Autodesk Inventor part; units mm, degrees
(part 2 of 2)
sketch "Sketch8" plane through (0, 0, 0) normal (0, 0, -1) x (-1, 0, 0)
  arc A0 (-1.4446, 6.1835) -> (1.4446, 6.1835) centre (0, 0) ccw construction
  circle A1 centre (0, 0) radius 44.45 construction
  spline S0 degree 2 poles (9.5387, -40.7098) (10.0629, -40.5828) (11.0086, -40.6927) (11.3992, -40.9412) knots 0 0 0 1 2 2 2
  spline S1 degree 2 poles (11.3992, -40.9412) (11.7907, -41.1937) (12.3573, -42.0815) (12.5094, -42.7097) knots 0 0 0 1 2 2 2
  spline S2 degree 2 poles (12.5094, -42.7097) (12.6538, -43.3058) (12.5463, -44.3315) (12.3156, -44.7431) knots 0 0 0 1 2 2 2
  spline S3 degree 2 poles (12.3156, -44.7431) (12.094, -45.1399) (11.2991, -45.7052) (10.7749, -45.8321) knots 0 0 0 1 2 2 2
  spline S4 degree 2 poles (10.7749, -45.8321) (10.5229, -45.8931) (10.0493, -45.9316) (9.8258, -45.9179) knots 0 0 0 1 2 2 2
  spline S5 degree 2 poles (9.8258, -45.9179) (9.6461, -45.9106) (9.1954, -45.8334) (9.0558, -45.7994) knots 0 0 0 1 2 2 2
  line L0 (9.0558, -45.7994) -> (8.864, -45.0072)
  line L1 (8.864, -45.0072) -> (8.92, -44.9936)
  spline S6 degree 2 poles (8.92, -44.9936) (9.0702, -45.0716) (9.3777, -45.2047) (9.6449, -45.2586) knots 0 0 0 1 2 2 2
  spline S7 degree 2 poles (9.6449, -45.2586) (9.8692, -45.3102) (10.4173, -45.3172) (10.7134, -45.2455) knots 0 0 0 1 2 2 2
  spline S8 degree 2 poles (10.7134, -45.2455) (11.4256, -45.0731) (12.0461, -43.7876) (11.8301, -42.8954) knots 0 0 0 1 2 2 2
  spline S9 degree 2 poles (11.8301, -42.8954) (11.7099, -42.3992) (11.2976, -41.7113) (11.0156, -41.5085) knots 0 0 0 1 2 2 2
  spline S10 degree 2 poles (11.0156, -41.5085) (10.7415, -41.3038) (10.0764, -41.181) (9.7003, -41.2721) knots 0 0 0 1 2 2 2
  spline S11 degree 2 poles (9.7003, -41.2721) (9.4243, -41.339) (8.8915, -41.5527) (8.7228, -41.6783) knots 0 0 0 1 2 2 2
  line L2 (8.7228, -41.6783) -> (9.0319, -42.9546)
  line L3 (9.0319, -42.9546) -> (10.1762, -42.6775)
  line L4 (10.1762, -42.6775) -> (10.3157, -43.2536)
  line L5 (10.3157, -43.2536) -> (8.5233, -43.6877)
  line L6 (8.5233, -43.6877) -> (8.001, -41.5311)
  spline S12 degree 2 poles (8.001, -41.5311) (8.1115, -41.4451) (8.4939, -41.1703) (8.6614, -41.0747) knots 0 0 0 1 2 2 2
  spline S13 degree 2 poles (8.6614, -41.0747) (8.888, -40.9436) (9.2627, -40.7766) (9.5387, -40.7098) knots 0 0 0 1 2 2 2
  spline S14 degree 2 poles (5.4812, -41.4638) (6.3864, -41.3379) (7.5225, -42.2148) (7.6529, -43.1527) knots 0 0 0 1 2 2 2
  spline S15 degree 2 poles (7.6529, -43.1527) (7.7811, -44.0742) (6.9667, -45.3013) (6.1879, -45.4096) knots 0 0 0 1 2 2 2
  spline S16 degree 2 poles (6.1879, -45.4096) (5.8372, -45.4584) (5.2666, -45.3299) (5.0367, -45.1416) knots 0 0 0 1 2 2 2
  spline S17 degree 2 poles (5.0367, -45.1416) (4.8028, -44.9538) (4.4999, -44.36) (4.437, -43.9074) knots 0 0 0 1 2 2 2
  line L7 (4.437, -43.9074) -> (4.3888, -43.5608)
  line L8 (4.3888, -43.5608) -> (7.0024, -43.1974)
  spline S18 degree 2 poles (7.0024, -43.1974) (6.9112, -42.5409) (6.1537, -41.9355) (5.5665, -42.0172) knots 0 0 0 1 2 2 2
  spline S19 degree 2 poles (5.5665, -42.0172) (5.3585, -42.0461) (4.9679, -42.196) (4.815, -42.2921) knots 0 0 0 1 2 2 2
  spline S20 degree 2 poles (4.815, -42.2921) (4.6551, -42.3974) (4.4385, -42.573) (4.3701, -42.6491) knots 0 0 0 1 2 2 2
  line L9 (4.3701, -42.6491) -> (4.3334, -42.6542)
  line L10 (4.3334, -42.6542) -> (4.237, -41.961)
  spline S21 degree 2 poles (4.237, -41.961) (4.3408, -41.9008) (4.657, -41.7239) (4.7824, -41.669) knots 0 0 0 1 2 2 2
  spline S22 degree 2 poles (4.7824, -41.669) (4.9585, -41.5905) (5.2529, -41.4955) (5.4812, -41.4638) knots 0 0 0 1 2 2 2
  spline S23 degree 2 poles (5.076, -43.9599) (5.1199, -44.2156) (5.2781, -44.576) (5.3976, -44.6882) knots 0 0 0 1 2 2 2
  spline S24 degree 2 poles (5.3976, -44.6882) (5.5276, -44.8156) (5.8951, -44.9183) (6.152, -44.8826) knots 0 0 0 1 2 2 2
  spline S25 degree 2 poles (6.152, -44.8826) (6.4048, -44.8474) (6.7386, -44.6472) (6.8649, -44.48) knots 0 0 0 1 2 2 2
  spline S26 degree 2 poles (6.8649, -44.48) (6.9867, -44.3093) (7.083, -43.926) (7.0699, -43.6826) knots 0 0 0 1 2 2 2
  line L11 (7.0699, -43.6826) -> (5.076, -43.9599)
  spline S27 degree 2 poles (1.3862, -42.2975) (1.4614, -42.236) (1.7141, -42.0171) (1.8343, -41.9491) knots 0 0 0 1 2 2 2
  spline S28 degree 2 poles (1.8343, -41.9491) (1.9983, -41.8501) (2.3101, -41.7395) (2.5979, -41.725) knots 0 0 0 1 2 2 2
  spline S29 degree 2 poles (2.5979, -41.725) (2.8322, -41.7131) (3.2647, -41.8684) (3.4331, -42.0207) knots 0 0 0 1 2 2 2
  spline S30 degree 2 poles (3.4331, -42.0207) (3.5932, -42.1692) (3.8015, -42.6203) (3.8144, -42.8752) knots 0 0 0 1 2 2 2
  spline S31 degree 2 poles (3.8144, -42.8752) (3.8344, -43.2699) (3.5297, -43.8459) (3.176, -44.0246) knots 0 0 0 1 2 2 2
  spline S32 degree 2 poles (3.176, -44.0246) (2.8628, -44.1889) (1.9968, -44.344) (1.4926, -44.3984) knots 0 0 0 1 2 2 2
  line L12 (1.4926, -44.3984) -> (1.4988, -44.5218)
  spline S33 degree 2 poles (1.4988, -44.5218) (1.5101, -44.7438) (1.6597, -45.0124) (1.787, -45.0842) knots 0 0 0 1 2 2 2
  spline S34 degree 2 poles (1.787, -45.0842) (1.9143, -45.1561) (2.2704, -45.1875) (2.4595, -45.1779) knots 0 0 0 1 2 2 2
  spline S35 degree 2 poles (2.4595, -45.1779) (2.6815, -45.1667) (3.2751, -45.0047) (3.5688, -44.8621) knots 0 0 0 1 2 2 2
  line L13 (3.5688, -44.8621) -> (3.6058, -44.8602)
  line L14 (3.6058, -44.8602) -> (3.6389, -45.5139)
  spline S36 degree 2 poles (3.6389, -45.5139) (3.4646, -45.5722) (2.809, -45.7291) (2.4841, -45.7455) knots 0 0 0 1 2 2 2
  spline S37 degree 2 poles (2.4841, -45.7455) (2.0895, -45.7655) (1.5446, -45.6695) (1.3227, -45.5199) knots 0 0 0 1 2 2 2
  spline S38 degree 2 poles (1.3227, -45.5199) (1.1051, -45.3743) (0.8743, -44.8873) (0.8562, -44.5296) knots 0 0 0 1 2 2 2
  line L15 (0.8562, -44.5296) -> (0.7244, -41.927)
  line L16 (0.7244, -41.927) -> (1.3658, -41.8946)
  line L17 (1.3658, -41.8946) -> (1.3862, -42.2975)
  line L18 (1.4132, -42.832) -> (1.4668, -43.8886)
  spline S39 degree 2 poles (1.4668, -43.8886) (1.696, -43.8564) (2.3873, -43.7513) (2.6018, -43.6745) knots 0 0 0 1 2 2 2
  spline S40 degree 2 poles (2.6018, -43.6745) (2.8528, -43.5834) (3.1693, -43.2418) (3.1548, -42.954) knots 0 0 0 1 2 2 2
  spline S41 degree 2 poles (3.1548, -42.954) (3.1381, -42.625) (2.7512, -42.3108) (2.3976, -42.3287) knots 0 0 0 1 2 2 2
  spline S42 degree 2 poles (2.3976, -42.3287) (2.0975, -42.3439) (1.6172, -42.6279) (1.4132, -42.832) knots 0 0 0 1 2 2 2
  line L19 (-2.2698, -44.9941) -> (-2.2369, -44.9948)
  spline S43 degree 2 poles (-2.2369, -44.9948) (-2.1633, -45.0171) (-2.0029, -45.0291) (-1.8918, -45.0316) knots 0 0 0 1 2 2 2
  spline S44 degree 2 poles (-1.8918, -45.0316) (-1.6325, -45.0377) (-1.117, -44.8231) (-0.8813, -44.6062) knots 0 0 0 1 2 2 2
  line L20 (-0.8813, -44.6062) -> (-0.8187, -41.9023)
  line L21 (-0.8187, -41.9023) -> (-0.1766, -41.9172)
  line L22 (-0.1766, -41.9172) -> (-0.265, -45.7282)
  line L23 (-0.265, -45.7282) -> (-0.907, -45.7133)
  line L24 (-0.907, -45.7133) -> (-0.8938, -45.1454)
  spline S45 degree 2 poles (-0.8938, -45.1454) (-1.2509, -45.45) (-1.7795, -45.6931) (-2.0264, -45.6874) knots 0 0 0 1 2 2 2
  spline S46 degree 2 poles (-2.0264, -45.6874) (-2.1252, -45.6851) (-2.2238, -45.6746) (-2.2852, -45.6608) knots 0 0 0 1 2 2 2
  line L25 (-2.2852, -45.6608) -> (-2.2698, -44.9941)
  line L26 (-8.8009, -41.0388) -> (-7.9348, -41.1759)
  line L27 (-7.9348, -41.1759) -> (-6.6649, -43.4233)
  line L28 (-6.6649, -43.4233) -> (-5.9005, -43.5442)
  line L29 (-5.9005, -43.5442) -> (-5.5846, -41.5478)
  line L30 (-5.5846, -41.5478) -> (-4.9177, -41.6533)
  line L31 (-4.9177, -41.6533) -> (-5.7117, -46.6709)
  line L32 (-5.7117, -46.6709) -> (-7.0047, -46.4662)
  spline S47 degree 2 poles (-7.0047, -46.4662) (-7.4357, -46.398) (-8.0024, -46.2125) (-8.2397, -45.9999) knots 0 0 0 1 2 2 2
  spline S48 degree 2 poles (-8.2397, -45.9999) (-8.4769, -45.7873) (-8.6976, -45.2064) (-8.6352, -44.812) knots 0 0 0 1 2 2 2
  spline S49 degree 2 poles (-8.6352, -44.812) (-8.5483, -44.2631) (-7.8695, -43.6078) (-7.3613, -43.5048) knots 0 0 0 1 2 2 2
  line L33 (-7.3613, -43.5048) -> (-8.8009, -41.0388)
  spline S50 degree 2 poles (-7.9315, -44.8692) (-7.9663, -45.0887) (-7.8652, -45.4507) (-7.7199, -45.5862) knots 0 0 0 1 2 2 2
  spline S51 degree 2 poles (-7.7199, -45.5862) (-7.5924, -45.7022) (-7.2264, -45.8393) (-6.9499, -45.8831) knots 0 0 0 1 2 2 2
  line L34 (-6.9499, -45.8831) -> (-6.2872, -45.9879)
  line L35 (-6.2872, -45.9879) -> (-5.9886, -44.1013)
  line L36 (-5.9886, -44.1013) -> (-6.5741, -44.0086)
  spline S52 degree 2 poles (-6.5741, -44.0086) (-6.8628, -43.9629) (-7.3384, -43.9919) (-7.5221, -44.1254) knots 0 0 0 1 2 2 2
  spline S53 degree 2 poles (-7.5221, -44.1254) (-7.6903, -44.2405) (-7.8903, -44.6089) (-7.9315, -44.8692) knots 0 0 0 1 2 2 2
  spline S54 degree 2 poles (-11.2959, -40.7848) (-11.2058, -40.7485) (-10.8993, -40.615) (-10.7642, -40.586) knots 0 0 0 1 2 2 2
  spline S55 degree 2 poles (-10.7642, -40.586) (-10.5782, -40.5405) (-10.2476, -40.5279) (-9.9686, -40.5999) knots 0 0 0 1 2 2 2
  spline S56 degree 2 poles (-9.9686, -40.5999) (-9.7413, -40.6585) (-9.375, -40.9357) (-9.2596, -41.1313) knots 0 0 0 1 2 2 2
  spline S57 degree 2 poles (-9.2596, -41.1313) (-9.1511, -41.3208) (-9.0869, -41.8135) (-9.1506, -42.0607) knots 0 0 0 1 2 2 2
  spline S58 degree 2 poles (-9.1506, -42.0607) (-9.2493, -42.4434) (-9.7119, -42.9022) (-10.1028, -42.9673) knots 0 0 0 1 2 2 2
  spline S59 degree 2 poles (-10.1028, -42.9673) (-10.4507, -43.0306) (-11.3236, -42.9203) (-11.8211, -42.8218) knots 0 0 0 1 2 2 2
  line L37 (-11.8211, -42.8218) -> (-11.8519, -42.9414)
  spline S60 degree 2 poles (-11.8519, -42.9414) (-11.9074, -43.1567) (-11.8448, -43.4577) (-11.7447, -43.5642) knots 0 0 0 1 2 2 2
  spline S61 degree 2 poles (-11.7447, -43.5642) (-11.6446, -43.6708) (-11.3142, -43.807) (-11.1308, -43.8543) knots 0 0 0 1 2 2 2
  spline S62 degree 2 poles (-11.1308, -43.8543) (-10.9155, -43.9098) (-10.3006, -43.9323) (-9.9778, -43.8838) knots 0 0 0 1 2 2 2
  line L38 (-9.9778, -43.8838) -> (-9.9419, -43.893)
  line L39 (-9.9419, -43.893) -> (-10.1053, -44.5269)
  spline S63 degree 2 poles (-10.1053, -44.5269) (-10.2891, -44.5305) (-10.9617, -44.4846) (-11.2766, -44.4034) knots 0 0 0 1 2 2 2
  spline S64 degree 2 poles (-11.2766, -44.4034) (-11.6593, -44.3047) (-12.1507, -44.0505) (-12.3179, -43.8416) knots 0 0 0 1 2 2 2
  spline S65 degree 2 poles (-12.3179, -43.8416) (-12.4821, -43.6377) (-12.5571, -43.104) (-12.4676, -42.7571) knots 0 0 0 1 2 2 2
  line L40 (-12.4676, -42.7571) -> (-11.817, -40.2338)
  line L41 (-11.817, -40.2338) -> (-11.1952, -40.3941)
  line L42 (-11.1952, -40.3941) -> (-11.2959, -40.7848)
  line L43 (-11.4295, -41.303) -> (-11.6937, -42.3275)
  spline S66 degree 2 poles (-11.6937, -42.3275) (-11.4653, -42.3651) (-10.7741, -42.4711) (-10.5464, -42.4618) knots 0 0 0 1 2 2 2
  spline S67 degree 2 poles (-10.5464, -42.4618) (-10.2797, -42.4497) (-9.8756, -42.2181) (-9.8037, -41.939) knots 0 0 0 1 2 2 2
  spline S68 degree 2 poles (-9.8037, -41.939) (-9.7215, -41.6201) (-9.997, -41.2047) (-10.3398, -41.1163) knots 0 0 0 1 2 2 2
  spline S69 degree 2 poles (-10.3398, -41.1163) (-10.6308, -41.0413) (-11.1739, -41.1691) (-11.4295, -41.303) knots 0 0 0 1 2 2 2
  spline S70 degree 2 poles (-13.7428, -39.5168) (-13.2471, -39.6833) (-12.8791, -40.4365) (-13.0848, -41.0492) knots 0 0 0 1 2 2 2
  line L44 (-13.0848, -41.0492) -> (-13.7571, -43.0512)
  line L45 (-13.7571, -43.0512) -> (-13.3473, -43.1888)
  line L46 (-13.3473, -43.1888) -> (-13.5164, -43.6923)
  line L47 (-13.5164, -43.6923) -> (-13.9261, -43.5547)
  line L48 (-13.9261, -43.5547) -> (-14.2747, -44.5927)
  line L49 (-14.2747, -44.5927) -> (-14.8835, -44.3883)
  line L50 (-14.8835, -44.3883) -> (-14.5349, -43.3502)
  line L51 (-14.5349, -43.3502) -> (-15.655, -42.9741)
  line L52 (-15.655, -42.9741) -> (-15.4859, -42.4707)
  line L53 (-15.4859, -42.4707) -> (-14.3659, -42.8468)
  line L54 (-14.3659, -42.8468) -> (-13.788, -41.1258)
  spline S71 degree 2 poles (-13.788, -41.1258) (-13.6962, -40.8526) (-13.6149, -40.5456) (-13.6379, -40.3945) knots 0 0 0 1 2 2 2
  spline S72 degree 2 poles (-13.6379, -40.3945) (-13.6546, -40.263) (-13.8624, -40.0672) (-14.0732, -39.9965) knots 0 0 0 1 2 2 2
  spline S73 degree 2 poles (-14.0732, -39.9965) (-14.2215, -39.9467) (-14.5287, -39.9434) (-14.6003, -39.9497) knots 0 0 0 1 2 2 2
  line L55 (-14.6003, -39.9497) -> (-14.6354, -39.938)
  line L56 (-14.6354, -39.938) -> (-14.452, -39.3916)
  spline S74 degree 2 poles (-14.452, -39.3916) (-14.2645, -39.4024) (-13.895, -39.4657) (-13.7428, -39.5168) knots 0 0 0 1 2 2 2
  line L57 (-15.4899, -38.9437) -> (-14.8914, -39.1765)
  line L58 (-14.8914, -39.1765) -> (-16.2731, -42.7293)
  line L59 (-16.2731, -42.7293) -> (-16.8716, -42.4966)
  line L60 (-16.8716, -42.4966) -> (-15.4899, -38.9437)
  line L61 (-17.1436, -43.071) -> (-16.4645, -43.3351)
  line L62 (-16.4645, -43.3351) -> (-16.7062, -43.9567)
  line L63 (-16.7062, -43.9567) -> (-17.3853, -43.6926)
  line L64 (-17.3853, -43.6926) -> (-17.1436, -43.071)
  spline S75 degree 2 poles (-20.0145, -39.0149) (-19.6084, -38.1414) (-18.326, -37.5799) (-17.6242, -37.9062) knots 0 0 0 1 2 2 2
  spline S76 degree 2 poles (-17.6242, -37.9062) (-16.9037, -38.2411) (-16.5351, -39.6064) (-16.9273, -40.4501) knots 0 0 0 1 2 2 2
  spline S77 degree 2 poles (-16.9273, -40.4501) (-17.3299, -41.3161) (-18.6271, -41.8798) (-19.3214, -41.5571) knots 0 0 0 1 2 2 2
  spline S78 degree 2 poles (-19.3214, -41.5571) (-20.0232, -41.2308) (-20.4189, -39.8847) (-20.0145, -39.0149) knots 0 0 0 1 2 2 2
  spline S79 degree 2 poles (-19.4135, -39.2943) (-19.7259, -39.9662) (-19.5406, -40.8468) (-19.0889, -41.0568) knots 0 0 0 1 2 2 2
  spline S80 degree 2 poles (-19.0889, -41.0568) (-18.6372, -41.2668) (-17.8407, -40.8426) (-17.5283, -40.1707) knots 0 0 0 1 2 2 2
  spline S81 degree 2 poles (-17.5283, -40.1707) (-17.2246, -39.5174) (-17.405, -38.6164) (-17.8567, -38.4064) knots 0 0 0 1 2 2 2
  spline S82 degree 2 poles (-17.8567, -38.4064) (-18.3047, -38.1981) (-19.1046, -38.6298) (-19.4135, -39.2943) knots 0 0 0 1 2 2 2
  line L65 (-22.195, -38.8607) -> (-21.4835, -39.2585)
  line L66 (-21.4835, -39.2585) -> (-21.9577, -40.1065)
  line L67 (-21.9577, -40.1065) -> (-22.6691, -39.7087)
  line L68 (-22.6691, -39.7087) -> (-22.195, -38.8607)
  line L69 (-20.8088, -36.3814) -> (-20.0973, -36.7792)
  line L70 (-20.0973, -36.7792) -> (-20.5714, -37.6272)
  line L71 (-20.5714, -37.6272) -> (-21.2829, -37.2294)
  line L72 (-21.2829, -37.2294) -> (-20.8088, -36.3814)
  spline S83 degree 2 poles (-27.5219, -37.4913) (-27.3729, -37.6015) (-27.0245, -37.7465) (-26.8406, -37.7955) knots 0 0 0 1 2 2 2
  spline S84 degree 2 poles (-26.8406, -37.7955) (-26.6665, -37.8372) (-26.3831, -37.8624) (-26.2679, -37.8658) knots 0 0 0 1 2 2 2
  line L73 (-26.2679, -37.8658) -> (-26.2348, -37.8902)
  line L74 (-26.2348, -37.8902) -> (-26.6631, -38.4695)
  spline S85 degree 2 poles (-26.6631, -38.4695) (-26.9128, -38.4333) (-27.6402, -38.136) (-27.9149, -37.9328) knots 0 0 0 1 2 2 2
  spline S86 degree 2 poles (-27.9149, -37.9328) (-28.193, -37.7272) (-28.5235, -37.3087) (-28.6042, -37.0647) knots 0 0 0 1 2 2 2
  spline S87 degree 2 poles (-28.6042, -37.0647) (-28.6874, -36.8034) (-28.5962, -36.2923) (-28.4101, -36.0408) knots 0 0 0 1 2 2 2
  spline S88 degree 2 poles (-28.4101, -36.0408) (-28.1605, -35.7032) (-27.34, -35.5215) (-26.9799, -35.6854) knots 0 0 0 1 2 2 2
  line L75 (-26.9799, -35.6854) -> (-26.9505, -35.6456)
  spline S89 degree 2 poles (-26.9505, -35.6456) (-27.06, -35.5237) (-27.2665, -35.1867) (-27.3041, -34.9745) knots 0 0 0 1 2 2 2
  spline S90 degree 2 poles (-27.3041, -34.9745) (-27.3442, -34.7656) (-27.229, -34.2774) (-27.0307, -34.0093) knots 0 0 0 1 2 2 2
  spline S91 degree 2 poles (-27.0307, -34.0093) (-26.8275, -33.7346) (-26.2937, -33.4075) (-25.9894, -33.356) knots 0 0 0 1 2 2 2
  spline S92 degree 2 poles (-25.9894, -33.356) (-25.6736, -33.3028) (-25.0252, -33.4854) (-24.7042, -33.7228) knots 0 0 0 1 2 2 2
  spline S93 degree 2 poles (-24.7042, -33.7228) (-24.3963, -33.9505) (-23.9041, -34.5449) (-23.7748, -34.7993) knots 0 0 0 1 2 2 2
  line L76 (-23.7748, -34.7993) -> (-24.2031, -35.3785)
  line L77 (-24.2031, -35.3785) -> (-24.2428, -35.3491)
  spline S94 degree 2 poles (-24.2428, -35.3491) (-24.3219, -35.0961) (-24.7331, -34.4336) (-25.0211, -34.2206) knots 0 0 0 1 2 2 2
  spline S95 degree 2 poles (-25.0211, -34.2206) (-25.1899, -34.0958) (-25.6058, -33.952) (-25.8089, -33.9913) knots 0 0 0 1 2 2 2
  spline S96 degree 2 poles (-25.8089, -33.9913) (-26.0087, -34.0329) (-26.34, -34.2385) (-26.504, -34.4603) knots 0 0 0 1 2 2 2
  spline S97 degree 2 poles (-26.504, -34.4603) (-26.668, -34.6821) (-26.7519, -35.0655) (-26.6972, -35.2339) knots 0 0 0 1 2 2 2
  spline S98 degree 2 poles (-26.6972, -35.2339) (-26.6426, -35.4023) (-26.3746, -35.6978) (-26.1893, -35.8348) knots 0 0 0 1 2 2 2
  line L78 (-26.1893, -35.8348) -> (-25.9576, -36.0062)
  line L79 (-25.9576, -36.0062) -> (-26.2929, -36.4596)
  line L80 (-26.2929, -36.4596) -> (-26.475, -36.325)
  spline S99 degree 2 poles (-26.475, -36.325) (-26.8424, -36.0533) (-27.5652, -36.0615) (-27.8125, -36.3958) knots 0 0 0 1 2 2 2
  spline S100 degree 2 poles (-27.8125, -36.3958) (-27.9275, -36.5513) (-27.9724, -36.8612) (-27.9253, -36.9984) knots 0 0 0 1 2 2 2
  spline S101 degree 2 poles (-27.9253, -36.9984) (-27.8741, -37.1438) (-27.6642, -37.3861) (-27.5219, -37.4913) knots 0 0 0 1 2 2 2
  line L81 (-27.6805, -31.4707) -> (-27.0633, -32.003)
  line L82 (-27.0633, -32.003) -> (-27.6978, -32.7387)
  line L83 (-27.6978, -32.7387) -> (-28.3151, -32.2064)
  line L84 (-28.3151, -32.2064) -> (-27.6805, -31.4707)
  line L85 (-29.5357, -33.6217) -> (-28.9185, -34.154)
  line L86 (-28.9185, -34.154) -> (-29.553, -34.8897)
  line L87 (-29.553, -34.8897) -> (-30.1702, -34.3574)
  line L88 (-30.1702, -34.3574) -> (-29.5357, -33.6217)
  line L89 (-30.6181, -28.6493) -> (-28.8678, -30.4038)
  line L90 (-28.8678, -30.4038) -> (-29.235, -30.7701)
  line L91 (-29.235, -30.7701) -> (-29.8863, -30.1173)
  line L92 (-29.8863, -30.1173) -> (-32.2965, -32.5218)
  line L93 (-32.2965, -32.5218) -> (-31.6452, -33.1746)
  line L94 (-31.6452, -33.1746) -> (-31.9746, -33.5031)
  spline S102 degree 2 poles (-31.9746, -33.5031) (-32.3438, -33.133) (-32.9025, -32.9926) (-33.2172, -33.26) knots 0 0 0 1 2 2 2
  line L95 (-33.2172, -33.26) -> (-33.5894, -32.887)
  line L96 (-33.5894, -32.887) -> (-30.3486, -29.6539)
  line L97 (-30.3486, -29.6539) -> (-30.9853, -29.0156)
  line L98 (-30.9853, -29.0156) -> (-30.6181, -28.6493)
  line L99 (-36.418, -26.5208) -> (-36.3978, -26.5468)
  spline S103 degree 2 poles (-36.3978, -26.5468) (-36.3689, -26.6181) (-36.2774, -26.7503) (-36.2096, -26.8383) knots 0 0 0 1 2 2 2
  spline S104 degree 2 poles (-36.2096, -26.8383) (-36.0512, -27.0437) (-35.5603, -27.3098) (-35.2435, -27.3567) knots 0 0 0 1 2 2 2
  line L100 (-35.2435, -27.3567) -> (-33.1013, -25.7056)
  line L101 (-33.1013, -25.7056) -> (-32.7092, -26.2142)
  line L102 (-32.7092, -26.2142) -> (-35.7285, -28.5414)
  line L103 (-35.7285, -28.5414) -> (-36.1206, -28.0327)
  line L104 (-36.1206, -28.0327) -> (-35.6706, -27.6859)
  spline S105 degree 2 poles (-35.6706, -27.6859) (-36.132, -27.5998) (-36.6534, -27.3415) (-36.8041, -27.1459) knots 0 0 0 1 2 2 2
  spline S106 degree 2 poles (-36.8041, -27.1459) (-36.8645, -27.0676) (-36.9183, -26.9843) (-36.9462, -26.9279) knots 0 0 0 1 2 2 2
  line L105 (-36.9462, -26.9279) -> (-36.418, -26.5208)
  spline S107 degree 2 poles (-35.0752, -22.782) (-34.5722, -23.5451) (-34.8753, -24.9479) (-35.6658, -25.469) knots 0 0 0 1 2 2 2
  spline S108 degree 2 poles (-35.6658, -25.469) (-36.4426, -25.981) (-37.9007, -25.7736) (-38.3335, -25.1171) knots 0 0 0 1 2 2 2
  spline S109 degree 2 poles (-38.3335, -25.1171) (-38.5283, -24.8215) (-38.6578, -24.251) (-38.5866, -23.9625) knots 0 0 0 1 2 2 2
  spline S110 degree 2 poles (-38.5866, -23.9625) (-38.5177, -23.6706) (-38.1119, -23.1418) (-37.7304, -22.8903) knots 0 0 0 1 2 2 2
  line L106 (-37.7304, -22.8903) -> (-37.4382, -22.6977)
  line L107 (-37.4382, -22.6977) -> (-35.986, -24.901)
  spline S111 degree 2 poles (-35.986, -24.901) (-35.4326, -24.5362) (-35.2119, -23.592) (-35.5381, -23.097) knots 0 0 0 1 2 2 2
  spline S112 degree 2 poles (-35.5381, -23.097) (-35.6537, -22.9217) (-35.957, -22.6335) (-36.1095, -22.5368) knots 0 0 0 1 2 2 2
  spline S113 degree 2 poles (-36.1095, -22.5368) (-36.2734, -22.4378) (-36.5251, -22.3177) (-36.6232, -22.2887) knots 0 0 0 1 2 2 2
  line L108 (-36.6232, -22.2887) -> (-36.6435, -22.2577)
  line L109 (-36.6435, -22.2577) -> (-36.0592, -21.8726)
  spline S114 degree 2 poles (-36.0592, -21.8726) (-35.9602, -21.9405) (-35.6645, -22.1498) (-35.561, -22.2394) knots 0 0 0 1 2 2 2
  spline S115 degree 2 poles (-35.561, -22.2394) (-35.4144, -22.3646) (-35.2021, -22.5895) (-35.0752, -22.782) knots 0 0 0 1 2 2 2
  spline S116 degree 2 poles (-37.5029, -23.4898) (-37.7149, -23.6394) (-37.9722, -23.9372) (-38.0221, -24.0934) knots 0 0 0 1 2 2 2
  spline S117 degree 2 poles (-38.0221, -24.0934) (-38.0813, -24.2655) (-38.0159, -24.6414) (-37.8731, -24.858) knots 0 0 0 1 2 2 2
  spline S118 degree 2 poles (-37.8731, -24.858) (-37.7327, -25.0711) (-37.4084, -25.2863) (-37.2031, -25.3285) knots 0 0 0 1 2 2 2
  spline S119 degree 2 poles (-37.2031, -25.3285) (-36.9966, -25.3649) (-36.6091, -25.287) (-36.395, -25.1706) knots 0 0 0 1 2 2 2
  line L110 (-36.395, -25.1706) -> (-37.5029, -23.4898)
  line L111 (-37.6144, -18.5405) -> (-37.3106, -19.1062)
  line L112 (-37.3106, -19.1062) -> (-37.6515, -19.2894)
  spline S120 degree 2 poles (-37.6515, -19.2894) (-37.4725, -19.3615) (-37.2242, -19.4758) (-37.0924, -19.5732) knots 0 0 0 1 2 2 2
  spline S121 degree 2 poles (-37.0924, -19.5732) (-36.9701, -19.6617) (-36.7702, -19.8861) (-36.6786, -20.0565) knots 0 0 0 1 2 2 2
  spline S122 degree 2 poles (-36.6786, -20.0565) (-36.5306, -20.3322) (-36.5097, -20.9191) (-36.6433, -21.2011) knots 0 0 0 1 2 2 2
  spline S123 degree 2 poles (-36.6433, -21.2011) (-36.7768, -21.4832) (-37.3322, -22.0151) (-37.7565, -22.243) knots 0 0 0 1 2 2 2
  spline S124 degree 2 poles (-37.7565, -22.243) (-38.199, -22.4807) (-38.9673, -22.599) (-39.3174, -22.53) knots 0 0 0 1 2 2 2
  spline S125 degree 2 poles (-39.3174, -22.53) (-39.6343, -22.4619) (-40.1631, -22.0777) (-40.317, -21.7912) knots 0 0 0 1 2 2 2
  spline S126 degree 2 poles (-40.317, -21.7912) (-40.4514, -21.541) (-40.5396, -21.1071) (-40.5346, -20.838) knots 0 0 0 1 2 2 2
  line L113 (-40.5346, -20.838) -> (-41.9853, -21.6172)
  line L114 (-41.9853, -21.6172) -> (-42.2892, -21.0515)
  line L115 (-42.2892, -21.0515) -> (-37.6144, -18.5405)
  line L116 (-38.1265, -19.5445) -> (-40.0668, -20.5867)
  spline S127 degree 2 poles (-40.0668, -20.5867) (-40.0554, -20.8516) (-39.9523, -21.2262) (-39.8491, -21.4184) knots 0 0 0 1 2 2 2
  spline S128 degree 2 poles (-39.8491, -21.4184) (-39.6153, -21.8536) (-38.6976, -21.9962) (-38.0811, -21.665) knots 0 0 0 1 2 2 2
  spline S129 degree 2 poles (-38.0811, -21.665) (-37.4863, -21.3455) (-37.0615, -20.6314) (-37.2855, -20.2143) knots 0 0 0 1 2 2 2
  spline S130 degree 2 poles (-37.2855, -20.2143) (-37.4043, -19.9931) (-37.849, -19.6525) (-38.1265, -19.5445) knots 0 0 0 1 2 2 2
  line L117 (-39.1721, -14.9731) -> (-38.9217, -15.5645)
  line L118 (-38.9217, -15.5645) -> (-39.3084, -15.7282)
  spline S131 degree 2 poles (-39.3084, -15.7282) (-38.954, -15.9) (-38.5006, -16.2848) (-38.3722, -16.588) knots 0 0 0 1 2 2 2
  spline S132 degree 2 poles (-38.3722, -16.588) (-38.2759, -16.8155) (-38.2558, -17.2853) (-38.3563, -17.5022) knots 0 0 0 1 2 2 2
  spline S133 degree 2 poles (-38.3563, -17.5022) (-38.4551, -17.7228) (-38.8811, -18.0999) (-39.2374, -18.2507) knots 0 0 0 1 2 2 2
  line L119 (-39.2374, -18.2507) -> (-41.5158, -19.2152)
  line L120 (-41.5158, -19.2152) -> (-41.7662, -18.6238)
  line L121 (-41.7662, -18.6238) -> (-39.7645, -17.7765)
  spline S134 degree 2 poles (-39.7645, -17.7765) (-39.484, -17.6577) (-39.1339, -17.4604) (-39.0279, -17.3306) knots 0 0 0 1 2 2 2
  spline S135 degree 2 poles (-39.0279, -17.3306) (-38.922, -17.2008) (-38.9012, -16.9014) (-38.9991, -16.6701) knots 0 0 0 1 2 2 2
  spline S136 degree 2 poles (-38.9991, -16.6701) (-39.0905, -16.454) (-39.544, -16.0693) (-39.8088, -15.94) knots 0 0 0 1 2 2 2
  line L122 (-39.8088, -15.94) -> (-42.4322, -17.0506)
  line L123 (-42.4322, -17.0506) -> (-42.6825, -16.4592)
  line L124 (-42.6825, -16.4592) -> (-39.1721, -14.9731)
  spline S137 degree 2 poles (-39.8725, -12.6306) (-39.7498, -13.0063) (-39.7775, -13.7039) (-39.9395, -14.0036) knots 0 0 0 1 2 2 2
  spline S138 degree 2 poles (-39.9395, -14.0036) (-40.0976, -14.3021) (-40.7293, -14.7812) (-41.2067, -14.937) knots 0 0 0 1 2 2 2
  spline S139 degree 2 poles (-41.2067, -14.937) (-41.6842, -15.0929) (-42.4638, -15.066) (-42.7689, -14.9274) knots 0 0 0 1 2 2 2
  spline S140 degree 2 poles (-42.7689, -14.9274) (-43.0779, -14.7901) (-43.5405, -14.2353) (-43.6606, -13.8674) knots 0 0 0 1 2 2 2
  spline S141 degree 2 poles (-43.6606, -13.8674) (-43.7577, -13.57) (-43.7709, -12.9594) (-43.7316, -12.7084) knots 0 0 0 1 2 2 2
  line L125 (-43.7316, -12.7084) -> (-43.0467, -12.4848)
  line L126 (-43.0467, -12.4848) -> (-43.0352, -12.52)
  spline S142 degree 2 poles (-43.0352, -12.52) (-43.0683, -12.6044) (-43.1427, -12.8539) (-43.1698, -13.023) knots 0 0 0 1 2 2 2
  spline S143 degree 2 poles (-43.1698, -13.023) (-43.1903, -13.1725) (-43.1757, -13.5489) (-43.1246, -13.7054) knots 0 0 0 1 2 2 2
  spline S144 degree 2 poles (-43.1246, -13.7054) (-42.97, -14.1789) (-42.066, -14.5204) (-41.4125, -14.307) knots 0 0 0 1 2 2 2
  spline S145 degree 2 poles (-41.4125, -14.307) (-40.7746, -14.0987) (-40.2399, -13.3092) (-40.4008, -12.8161) knots 0 0 0 1 2 2 2
  spline S146 degree 2 poles (-40.4008, -12.8161) (-40.498, -12.5187) (-40.9208, -12.0591) (-41.1803, -11.9143) knots 0 0 0 1 2 2 2
  line L127 (-41.1803, -11.9143) -> (-41.1918, -11.8791)
  line L128 (-41.1918, -11.8791) -> (-40.5069, -11.6555)
  spline S147 degree 2 poles (-40.5069, -11.6555) (-40.4345, -11.7315) (-40.2238, -11.9658) (-40.1606, -12.0664) knots 0 0 0 1 2 2 2
  spline S148 degree 2 poles (-40.1606, -12.0664) (-40.0625, -12.2076) (-39.9351, -12.4389) (-39.8725, -12.6306) knots 0 0 0 1 2 2 2
  spline S149 degree 2 poles (-40.6537, -9.8854) (-40.5247, -10.3921) (-40.958, -11.1098) (-41.5843, -11.2693) knots 0 0 0 1 2 2 2
  line L129 (-41.5843, -11.2693) -> (-43.6309, -11.7903)
  line L130 (-43.6309, -11.7903) -> (-43.5243, -12.2091)
  line L131 (-43.5243, -12.2091) -> (-44.0389, -12.3401)
  line L132 (-44.0389, -12.3401) -> (-44.1456, -11.9213)
  line L133 (-44.1456, -11.9213) -> (-45.2067, -12.1914)
  line L134 (-45.2067, -12.1914) -> (-45.3652, -11.569)
  line L135 (-45.3652, -11.569) -> (-44.304, -11.2989)
  line L136 (-44.304, -11.2989) -> (-44.5954, -10.1539)
  line L137 (-44.5954, -10.1539) -> (-44.0808, -10.0229)
  line L138 (-44.0808, -10.0229) -> (-43.7893, -11.1679)
  line L139 (-43.7893, -11.1679) -> (-42.03, -10.72)
  spline S150 degree 2 poles (-42.03, -10.72) (-41.7507, -10.649) (-41.4486, -10.5508) (-41.3342, -10.4495) knots 0 0 0 1 2 2 2
  spline S151 degree 2 poles (-41.3342, -10.4495) (-41.2327, -10.3642) (-41.181, -10.0834) (-41.2359, -9.868) knots 0 0 0 1 2 2 2
  spline S152 degree 2 poles (-41.2359, -9.868) (-41.2744, -9.7164) (-41.4383, -9.4565) (-41.4825, -9.3997) knots 0 0 0 1 2 2 2
  line L140 (-41.4825, -9.3997) -> (-41.4916, -9.3638)
  line L141 (-41.4916, -9.3638) -> (-40.9331, -9.2217)
  spline S153 degree 2 poles (-40.9331, -9.2217) (-40.8405, -9.385) (-40.6933, -9.7299) (-40.6537, -9.8854) knots 0 0 0 1 2 2 2
  line L142 (-41.1197, -8.1068) -> (-40.9907, -8.7359)
  line L143 (-40.9907, -8.7359) -> (-44.725, -9.5018)
  line L144 (-44.725, -9.5018) -> (-44.854, -8.8727)
  line L145 (-44.854, -8.8727) -> (-41.1197, -8.1068)
  line L146 (-45.4842, -8.9558) -> (-45.3378, -9.6696)
  line L147 (-45.3378, -9.6696) -> (-45.9911, -9.8036)
  line L148 (-45.9911, -9.8036) -> (-46.1375, -9.0898)
  line L149 (-46.1375, -9.0898) -> (-45.4842, -8.9558)
  spline S154 degree 2 poles (-43.6334, -4.3439) (-42.6792, -4.2114) (-41.512, -4.9843) (-41.4055, -5.7509) knots 0 0 0 1 2 2 2
  spline S155 degree 2 poles (-41.4055, -5.7509) (-41.2962, -6.5379) (-42.2433, -7.588) (-43.1649, -7.716) knots 0 0 0 1 2 2 2
  spline S156 degree 2 poles (-43.1649, -7.716) (-44.1108, -7.8475) (-45.2879, -7.0634) (-45.3933, -6.305) knots 0 0 0 1 2 2 2
  spline S157 degree 2 poles (-45.3933, -6.305) (-45.4998, -5.5384) (-44.5834, -4.4759) (-43.6334, -4.3439) knots 0 0 0 1 2 2 2
  spline S158 degree 2 poles (-43.5422, -5.0004) (-44.2761, -5.1024) (-44.9155, -5.7357) (-44.8469, -6.2291) knots 0 0 0 1 2 2 2
  spline S159 degree 2 poles (-44.8469, -6.2291) (-44.7784, -6.7224) (-43.99, -7.1615) (-43.2561, -7.0596) knots 0 0 0 1 2 2 2
  spline S160 degree 2 poles (-43.2561, -7.0596) (-42.5425, -6.9604) (-41.8833, -6.3202) (-41.9519, -5.8268) knots 0 0 0 1 2 2 2
  spline S161 degree 2 poles (-41.9519, -5.8268) (-42.0199, -5.3375) (-42.8164, -4.8996) (-43.5422, -5.0004) knots 0 0 0 1 2 2 2
  line L150 (-41.935, -0.4359) -> (-41.9052, -1.0774)
  line L151 (-41.9052, -1.0774) -> (-44.0764, -1.1783)
  spline S162 degree 2 poles (-44.0764, -1.1783) (-44.3396, -1.1905) (-44.7897, -1.2609) (-44.9219, -1.3412) knots 0 0 0 1 2 2 2
  spline S163 degree 2 poles (-44.9219, -1.3412) (-45.0622, -1.426) (-45.1891, -1.7122) (-45.178, -1.9507) knots 0 0 0 1 2 2 2
  spline S164 degree 2 poles (-45.178, -1.9507) (-45.1669, -2.1892) (-44.8884, -2.6831) (-44.6715, -2.9162) knots 0 0 0 1 2 2 2
  line L152 (-44.6715, -2.9162) -> (-41.8259, -2.784)
  line L153 (-41.8259, -2.784) -> (-41.7961, -3.4255)
  line L154 (-41.7961, -3.4255) -> (-45.604, -3.6024)
  line L155 (-45.604, -3.6024) -> (-45.6338, -2.9609)
  line L156 (-45.6338, -2.9609) -> (-45.2103, -2.9412)
  spline S165 degree 2 poles (-45.2103, -2.9412) (-45.4827, -2.6654) (-45.7799, -2.1229) (-45.7944, -1.8103) knots 0 0 0 1 2 2 2
  spline S166 degree 2 poles (-45.7944, -1.8103) (-45.8204, -1.2511) (-45.1096, -0.5834) (-44.4064, -0.5507) knots 0 0 0 1 2 2 2
  line L157 (-44.4064, -0.5507) -> (-41.935, -0.4359)
  dimension "d38" = 88.9
  constraints: 1 centre point, 1 coincident, 1 other
  measures "d38" diameter of A1
extrude "Extrusion6" cut sketch "Sketch8" against normal blind 3.175
sketch "Sketch9" plane through (0, 0, -22.098) normal (0, 0, -1) x (-1, 0, 0)
  circle A0 centre (0, 0) radius 5.0165
  dimension "d44" = 10.033
  constraints: 1 centre point, 1 coincident
  measures "d44" diameter of A0
extrude "Extrusion7" cut sketch "Sketch9" against normal through all
equation "\"d0\" = da_da"
equation "\"d1\" = da_b"
equation "\"d3\" = da_dw"
equation "\"d15\" = da_aw"
equation "\"d19\" = da_aw"
equation "\"da_da\" = 110.303074"
equation "\"da_b\" = 9.525"
equation "\"da_dw\" = 107.763074"
equation "\"da_aw\" = 71.842049"
body "Solid1"
body "Srf1"
